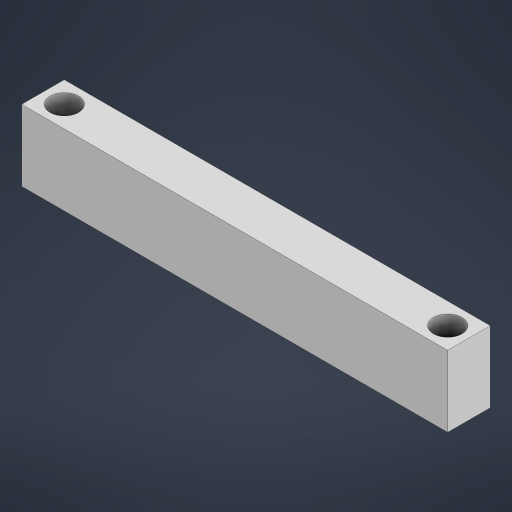
# Autodesk Inventor part: link
Saved by Autodesk Inventor 2024.3 (Build 283343000, 343)
## iProperties
Created: 2024-09-28
Part Number: link
Material: Generic
Document SubType Name: Modeling
Designer: sam
Density: 1 g/cm^3
Appearance: Default
Author: sam
Autodesk Inventor part; units mm, degrees
ref_plane "YZ Plane" through (0, 0, 0) normal (1, 0, 0) x (0, 1, 0)
ref_plane "XZ Plane" through (0, 0, 0) normal (0, 1, 0) x (-1, 0, 0)
ref_plane "XY Plane" through (0, 0, 0) normal (0, 0, 1) x (1, 0, 0)
sketch "Sketch1" plane through (0, 0, 0) normal (0, 1, 0) x (-1, 0, 0)
  line L0 (-15, -1.5) -> (15, -1.5)
  line L1 (15, 3.5) -> (15, 3.5)
  line L2 (15, 1.5) -> (-15, 1.5)
  line L3 (-15, 3.5) -> (-15, 3.5)
  line L4 (-15, -1.5) -> (15, 1.5) construction
  line L5 (15, -1.5) -> (-15, 1.5) construction
  circle A0 centre (13.5, 0) radius 1
  line L6 (-15, 1.5) -> (-15, -1.5)
  line L7 (15, 1.5) -> (15, -1.5)
  circle A1 centre (-13.5, 0) radius 1
  point P0 (0, 0)
  dimension "d0" = 3
  dimension "d1" = 30
  dimension "d3" = 2
  dimension "d6" = 1.5
  dimension "d8" = 1.5
  dimension "d13" = 2
  dimension "d14" = 1.5
  dimension "d15" = 1.5
  constraints: 16 end point, 4 point on line, 3 perpendicular, 2 centre point, 2 midpoint, 2 parallel, 1 horizontal
  measures "d0" distance of L2.start L0.end
  measures "d1" distance between parallel lines of L3 L1
  measures "d3" diameter of A0
  measures "d6" distance from line of L1 A0.centre
  measures "d8" distance from line of L2 A0.centre
  measures "d13" diameter of A1
  measures "d14" distance from line of L6 A1.centre
  measures "d15" distance from line of L2 A1.centre
extrude "Extrusion1" add sketch "Sketch1" along normal blind 5
body "Solid1"
